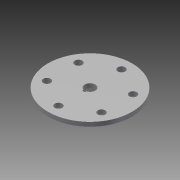
# Autodesk Inventor part: Hub v1
Saved by Autodesk Inventor 2013 (Build 170138000, 138)
## iProperties
Created: 2013-01-16
Part Number: Hub v1
Material: Steel
Document SubType Name: Modeling
Designer: actoennies
Mass: 73.9599 g
Surface Area: 69.8954 cm^2
Volume: 9.42164 cm^3
Density: 7.85 g/cm^3
Author: actoennies
Autodesk Inventor part; units mm, degrees
ref_plane "YZ Plane" through (0, 0, 0) normal (1, 0, 0) x (0, 1, 0)
ref_plane "XZ Plane" through (0, 0, 0) normal (0, 1, 0) x (-1, 0, 0)
ref_plane "XY Plane" through (0, 0, 0) normal (0, 0, 1) x (1, 0, 0)
sketch "Sketch1" plane through (0, 0, 0) normal (0, 1, 0) x (-1, 0, 0)
  circle A0 centre (0, 0) radius 31.75
  circle A1 centre (0, -23.8125) radius 2.794
  circle A2 centre (20.6222, -11.9063) radius 2.794
  circle A3 centre (20.6222, 11.9062) radius 2.794
  circle A4 centre (0, 23.8125) radius 2.794
  circle A5 centre (-20.6222, 11.9062) radius 2.794
  circle A6 centre (-20.6222, -11.9063) radius 2.794
  line L0 (2.7496, 4.7625) -> (5.4993, 0)
  line L1 (5.4993, 0) -> (2.7496, -4.7625)
  line L2 (2.7496, -4.7625) -> (-2.7496, -4.7625)
  line L3 (-2.7496, -4.7625) -> (-5.4993, 0)
  line L4 (-5.4993, 0) -> (-2.7496, 4.7625)
  line L5 (-2.7496, 4.7625) -> (2.7496, 4.7625)
  line L6 (0, 0) -> (0, -23.8125) construction
  dimension "d5" = 5.588
  dimension "d9" = 360
  dimension "d22" = 9.525
  dimension "d25" = 23.8125
  constraints: 14 end point, 7 centre point, 1 coincident, 1 perpendicular, 1 vertical, 27 other
  measures "d5" diameter of A1
  measures "d22" distance between parallel lines of L2 L5
  measures "d25" distance of A0.centre L6.end
extrude "Extrusion3" add sketch "Sketch1" along normal blind 3.175
sketch "Sketch3" plane through (0, 0, 0) normal (0, -1, 0) x (1, 0, 0)
  circle A0 centre (20.6222, -11.9063) radius 2.794 projected
  circle A1 centre (20.6222, 11.9062) radius 2.794 projected
  circle A2 centre (0, 23.8125) radius 2.794 projected
  circle A3 centre (-20.6222, 11.9062) radius 2.794 projected
  circle A4 centre (-20.6222, -11.9063) radius 2.794 projected
  circle A5 centre (0, -23.8125) radius 2.794 projected
  circle A6 centre (0, 0) radius 31.75 projected
  circle A7 centre (0, 0) radius 4
  dimension "d26" = 8
  constraints: 1 centre point, 1 coincident
  measures "d26" diameter of A7
extrude "Extrusion4" add sketch "Sketch3" against normal blind 3.175
sketch "Sketch4" plane through (0, 0, 0) normal (0, -1, 0) x (1, 0, 0)
  circle A0 centre (0, 0) radius 4 projected
  line L0 (-1, 3.873) -> (-1, 5)
  line L1 (-1, 5) -> (1, 5)
  line L2 (1, 5) -> (1, 3.873)
  dimension "d29" = 1
  dimension "d30" = 1
  dimension "d31" = 5
  constraints: 6 end point, 2 point on circle, 1 parallel, 1 perpendicular, 1 vertical
  measures "d29" distance from line of L2 A0.centre
  measures "d30" distance from line of A0.centre L0
  measures "d31" distance from line of A0.centre L1
extrude "Extrusion5" cut sketch "Sketch4" against normal blind 3.175 contours A0 L0 L1 L2
body "Solid3"
